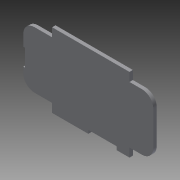
# Autodesk Inventor part: kryt_novy
Saved by Autodesk Inventor 2015 (Build 190159000, 159)
## iProperties
Created: 2015-10-21
Part Number: kryt_novy
Material: Generic
Document SubType Name: Modeling
Designer: Turboslimak
Density: 1 g/cm^3
Appearance: Default
Author: Turboslimak
Autodesk Inventor part; units mm, degrees
ref_plane "YZ Plane" through (0, 0, 0) normal (1, 0, 0) x (0, 1, 0)
ref_plane "XZ Plane" through (0, 0, 0) normal (0, 1, 0) x (-1, 0, 0)
ref_plane "XY Plane" through (0, 0, 0) normal (0, 0, 1) x (1, 0, 0)
sketch "Sketch1" plane through (0, 0, 0) normal (0, 1, 0) x (-1, 0, 0)
  line L0 (-115, -50.2) -> (-72.8, -50.2)
  line L1 (-72.8, -50.2) -> (-72.8, -65.6)
  line L2 (-115, 50.2) -> (-72.8, 50.2)
  line L3 (-72.8, 50.2) -> (-72.8, 65.6)
  line L4 (-72.8, -50.2) -> (-72.8, -65.6)
  line L5 (-72.8, 50.2) -> (-72.8, 65.6)
  line L6 (-72.8, 65.6) -> (-72.8, 62.6)
  line L7 (115, 50.2) -> (115, 10.2)
  line L8 (115, 10.2) -> (112, 10.2)
  line L9 (112, 10.2) -> (112, -20.2)
  line L10 (112, -20.2) -> (115, -20.2)
  line L11 (115, -20.2) -> (115, -50.2)
  line L12 (-115, -50.2) -> (-115, 50.2)
  line L13 (115, 50.2) -> (115, 10.2)
  line L14 (115, 10.2) -> (112, 10.2)
  line L15 (112, 10.2) -> (112, -20.2)
  line L16 (112, -20.2) -> (115, -20.2)
  line L17 (115, -20.2) -> (115, -50.2)
  line L18 (-72.8, -65.6) -> (-72.8, -50.2)
  line L19 (-72.8, -50.2) -> (-115, -50.2)
  line L20 (-115, -50.2) -> (-115, 50.2)
  line L21 (-115, 50.2) -> (-72.8, 50.2)
  line L22 (-72.8, 50.2) -> (-72.8, 65.6)
  line L23 (115, 50.2) -> (64, 50.2)
  line L24 (64, 50.2) -> (64, 65.6)
  line L25 (64, -50.2) -> (64, -65.6)
  line L26 (115, -50.2) -> (64, -50.2)
  line L27 (64, -50.2) -> (64, -65.6)
  line L28 (0, -65.6) -> (6, -65.6) construction
  line L29 (0, -59.6) -> (-50, -59.6)
  line L30 (64, -65.6) -> (0, -65.6)
  line L31 (0, -65.6) -> (0, -59.6)
  line L32 (-50, -59.6) -> (-50, -65.6)
  line L33 (-50, -65.6) -> (-72.8, -65.6)
  line L34 (64, 65.6) -> (-72.8, 65.6)
  point P0 (0, 0)
  dimension "d0" = 230
  dimension "d1" = 100.4
  dimension "d2" = 42.2
  dimension "d3" = 15.4
  dimension "d4" = 42.2
  dimension "d5" = 15.4
  dimension "d13" = 40
  dimension "d14" = 3
  dimension "d15" = 30.4
  dimension "d21" = 6
  constraints: 70 end point, 8 perpendicular, 7 collinear, 5 horizontal, 2 vertical, 1 parallel, 1 point on line
  measures "d0" distance of L7.start L2.start
  measures "d1" distance of L11.end L7.start
  measures "d2" distance of L0.start L0.end
  measures "d3" distance of L0.end L1.end
  measures "d4" distance of L2.start L2.end
  measures "d5" distance of L2.end L3.end
  measures "d13" distance of L7.start L7.end
  measures "d14" distance of L7.end L8.end
  measures "d15" distance of L8.end L9.end
  measures "d21" distance of L28.start L29.start
extrude "Extrusion1" add sketch "Sketch1" along normal blind 6
fillet "Fillet1" radius 20 4 edges at (115, 3, 50.2) (115, 3, -50.2) (-115, 3, -50.2) (-115, 3, 50.2)
body "Solid1"
